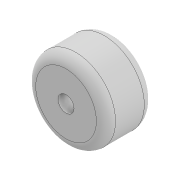
# Autodesk Inventor part: castor_wheel
Saved by Autodesk Inventor 2020 (Build 240168000, 168)
## iProperties
Created: 2020-09-08
Part Number: castor_wheel
Material: 일반
Document SubType Name: Modeling
Designer: 이호석
Mass: 6.78146 g
Surface Area: 21.4593 cm^2
Volume: 6.78146 cm^3
Density: 1 g/cm^3
Appearance: 기본값
Author: 이호석
Autodesk Inventor part; units mm, degrees
ref_plane "YZ Plane" through (0, 0, 0) normal (1, 0, 0) x (0, 1, 0)
ref_plane "XZ Plane" through (0, 0, 0) normal (0, 1, 0) x (-1, 0, 0)
ref_plane "XY Plane" through (0, 0, 0) normal (0, 0, 1) x (1, 0, 0)
sketch "스케치1" plane through (0, 0, 0) normal (0, 0, 1) x (1, 0, 0)
  circle A0 centre (0, 0) radius 12.5
  circle A1 centre (0, 0) radius 2.5
  dimension "d0" = 25
  dimension "d1" = 5
  constraints: 2 centre point, 2 coincident
  measures "d0" diameter of A0
  measures "d1" diameter of A1
extrude "돌출1" add sketch "스케치1" along normal blind 15
fillet "모깎기1" radius 3 2 edges at (-12.5, 0, 15) (-12.5, 0, 0)
